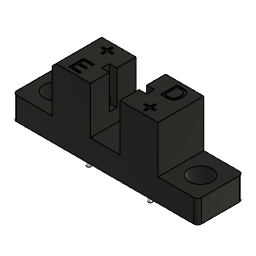
MOC7811 (Autodesk Fusion 360 design; units mm, degrees)
Autodesk Fusion 360 part; units mm, degrees
sketch "Sketch2" plane through (0, 0, 0) normal (0, 1, 0) x (1, 0, 0)
  line L0 (0, 0) -> (24.3, 0)
  line L1 (24.3, 0) -> (24.3, -3)
  line L2 (24.3, -3) -> (19.1, -3)
  line L3 (19.1, -3) -> (19.1, -9.2)
  line L4 (19.1, -9.2) -> (14.1, -9.2)
  line L5 (14.1, -9.2) -> (14.1, -3)
  line L6 (14.1, -3) -> (10.2, -3)
  line L7 (10.2, -3) -> (10.2, -9.2)
  line L8 (10.2, -9.2) -> (5.2, -9.2)
  line L9 (5.2, -9.2) -> (5.2, -3)
  line L10 (5.2, -3) -> (0, -3)
  line L11 (0, -3) -> (0, 0)
  dimension "d1" = 24.3
  dimension "d2" = 3
  dimension "d4" = 6.2
  dimension "d5" = 5
  dimension "d6" = 6.2
  dimension "d7" = 3.9
  dimension "d8" = 6.2
  dimension "d9" = 5
  dimension "d10" = 6.2
  constraint coincident L0.start L11.end
  constraint horizontal L0
  constraint perpendicular L0 L1
  constraint perpendicular L1 L2
  constraint perpendicular L2 L3
  constraint perpendicular L3 L4
  constraint perpendicular L4 L5
  constraint perpendicular L5 L6
  constraint perpendicular L6 L7
  constraint perpendicular L7 L8
  constraint perpendicular L8 L9
  constraint perpendicular L7 L10
  constraint perpendicular L0 L11
  constraint equal L2 L10
  measures "d1" distance of L0.start L0.end
  measures "d2" distance of L0.end L1.end
  measures "d4" distance of L2.end L3.end
  measures "d5" distance of L3.end L4.end
  measures "d6" distance of L4.end L5.end
  measures "d7" distance of L5.end L6.end
  measures "d8" distance of L6.end L7.end
  measures "d9" distance of L7.end L8.end
  measures "d10" distance of L8.end L9.end
extrude "Extrude1" add sketch "Sketch2" along normal blind 6
sketch "Sketch3" plane through (0, 0, 3) normal (0, 0, 1) x (-1, 0, 0)
  line L0 (0, 0) -> (-5.2, 0)
  line L1 (-5.2, 0) -> (-5.2, -6)
  line L2 (-5.2, -6) -> (0, -6)
  line L3 (0, -6) -> (0, 0)
  line L4 (-5.2, -6) -> (0, 0) construction
  line L5 (-5.2, 0) -> (0, -6) construction
  circle A0 centre (-2.6, -3) radius 1.5
  dimension "d13" = 3
  constraint coincident L1.end L2.start
  constraint coincident L0.start L3.end
  constraint coincident L0.end L1.start
  constraint coincident L2.end L3.start
  constraint midpoint L4 A0.centre
  measures "d13" diameter of A0
extrude "Extrude2" cut sketch "Sketch3" against normal blind 3 contours A0
sketch "Sketch4" plane through (0, 0, 3) normal (0, 0, 1) x (-1, 0, 0)
  line L0 (-19.1, 0) -> (-24.3, 0)
  line L1 (-24.3, 0) -> (-24.3, -6)
  line L2 (-24.3, -6) -> (-19.1, -6)
  line L3 (-19.1, -6) -> (-19.1, 0)
  line L4 (-19.1, -6) -> (-24.3, 0) construction
  line L5 (-24.3, -6) -> (-19.1, 0) construction
  circle A0 centre (-21.7, -3) radius 1.5
  dimension "d16" = 3
  constraint coincident L2.end L3.start
  constraint coincident L0.end L1.start
  constraint coincident L1.end L2.start
  constraint coincident L0.start L3.end
  constraint midpoint L4 A0.centre
  measures "d16" diameter of A0
extrude "Extrude3" cut sketch "Sketch4" against normal blind 3 contours A0
chamfer "Chamfer1" distance 0.5 angle 45 1 edges at (5.2, 3, 9.2)
sketch "Sketch5" plane through (10.2, 0, 0) normal (1, 0, 0) x (0, 1, 0)
  line L0 (0, 9.2) -> (0, 3)
  line L1 (0, 3) -> (6, 3)
  line L2 (6, 3) -> (6, 9.2)
  line L3 (6, 9.2) -> (0, 9.2)
fillet "Fillet1" radius 0.5 2 edges at (0, 6, 1.5) (0, 0, 1.5)
fillet "Fillet2" radius 0.5 2 edges at (24.3, 0, 1.5) (24.3, 6, 1.5)
sketch "Sketch7" plane through (0, 0, 9.2) normal (0, 0, 1) x (-1, 0, 0)
  line L0 (-5.7, -6) -> (-5.7, 0)
  line L1 (-5.7, 0) -> (-10.2, 0)
  line L2 (-10.2, 0) -> (-10.2, -6)
  line L3 (-10.2, -6) -> (-5.7, -6)
  line L4 (-11.2, -2.5) -> (-9.2, -2.5)
  line L5 (-9.2, -2.5) -> (-9.2, -3.5)
  line L6 (-9.2, -3.5) -> (-11.2, -3.5)
  line L7 (-11.2, -3.5) -> (-11.2, -2.5)
  line L8 (-11.2, -2.5) -> (-9.2, -3.5) construction
  line L9 (-9.2, -2.5) -> (-11.2, -3.5) construction
  point P0 (-10.2, -3)
  dimension "d22" = 2
  dimension "d23" = 1
  constraint horizontal L4
  constraint perpendicular L4 L5
  constraint parallel L4 L6
  constraint parallel L5 L7
  constraint coincident L8 P0
  constraint coincident L9 P0
  constraint midpoint L2 P0
  measures "d22" distance of L5.end L6.end
  measures "d23" distance of L4.end L5.end
extrude "Extrude4" cut sketch "Sketch7" against normal blind 4.5 contours L2 L4 L5 L6
ref_plane "WorkPlane1" through (12.15, 3, 5.85) normal (-1, 0, 0) x (0, 0, 1)
mirror "Mirror1" about plane through (12.15, 3, 5.85) normal (-1, 0, 0) of 4 faces at (9.5333, 3.5, 7.7) (9.2, 2.8333, 7.7) (9.8667, 2.5, 7.7) (9.5333, 3.1667, 4.7)
sketch "Sketch8" plane through (0, 0, 0) normal (0, 0, -1) x (1, 0, 0)
  arc A0 (23.8, -6) -> (24.3, -5.5) centre (23.8, -5.5) ccw
  line L0 (24.3, -5.5) -> (24.3, -0.5)
  arc A1 (24.3, -0.5) -> (23.8, 0) centre (23.8, -0.5) ccw
  line L1 (23.8, 0) -> (0.5, 0)
  arc A2 (0.5, 0) -> (0, -0.5) centre (0.5, -0.5) ccw
  line L2 (0, -0.5) -> (0, -5.5)
  arc A3 (0, -5.5) -> (0.5, -6) centre (0.5, -5.5) ccw
  line L3 (0.5, -6) -> (23.8, -6)
  circle A4 centre (21.7, -3) radius 1.5
  circle A5 centre (2.6, -3) radius 1.5
  line L4 (17.3061, -5.5) -> (7.3061, -5.5)
  line L5 (7.3061, -5.5) -> (7.3061, -0.5)
  line L6 (7.3061, -0.5) -> (17.3061, -0.5)
  line L7 (17.3061, -0.5) -> (17.3061, -5.5)
  line L8 (17.3061, -5.5) -> (7.3061, -0.5) construction
  line L9 (7.3061, -5.5) -> (17.3061, -0.5) construction
  point P0 (12.3061, -3)
  dimension "d27" = 10
  dimension "d28" = 5
  constraint horizontal L4
  constraint perpendicular L4 L5
  constraint parallel L4 L6
  constraint parallel L5 L7
  constraint coincident L8 P0
  constraint coincident L9 P0
  measures "d27" distance of L5.end L6.end
  measures "d28" distance of L4.end L5.end
extrude "Extrude5" cut sketch "Sketch8" against normal blind 2 contours L4 L5 L6 L7
sketch "Sketch9" plane through (0, 0, 2) normal (0, 0, -1) x (1, 0, 0)
  line L0 (17.3061, -0.5) -> (7.3061, -0.5)
  line L1 (7.3061, -0.5) -> (7.3061, -5.5)
  line L2 (7.3061, -5.5) -> (17.3061, -5.5)
  line L3 (17.3061, -5.5) -> (17.3061, -0.5)
  line L4 (7.3061, -0.5) -> (9.3061, -0.5)
  line L5 (9.3061, -0.5) -> (9.3061, -5.5)
  line L6 (9.3061, -5.5) -> (7.3061, -5.5)
  line L7 (7.3061, -5.5) -> (7.3061, -0.5)
  line L8 (17.3061, -0.5) -> (15.3061, -0.5)
  line L9 (15.3061, -0.5) -> (15.3061, -6)
  line L10 (15.3061, -6) -> (17.3061, -6)
  line L11 (17.3061, -6) -> (17.3061, -0.5)
  dimension "d31" = 2
  dimension "d32" = 2
  constraint horizontal L4
  constraint vertical L5
  constraint horizontal L6
  constraint vertical L7
  constraint coincident L0.end L1.start
  constraint horizontal L8
  constraint vertical L9
  constraint horizontal L10
  constraint vertical L11
  constraint coincident L0.start L3.end
  measures "d31" distance of L0.end L4.end
  measures "d32" distance of L0.start L8.end
extrude "Extrude6" cut sketch "Sketch9" against normal blind 3.5 contours L0 L2 L3 L8 L9 L11 | L0 L1 L2 L4 L5 L6 L7
sketch "Sketch10" plane through (0, 0, 5.5) normal (0, 0, -1) x (1, 0, 0)
  line L0 (9.3061, -3.5) -> (9.2, -3.5)
  line L1 (9.2, -3.5) -> (9.2, -2.5)
  line L2 (9.2, -2.5) -> (9.3061, -2.5)
  line L3 (9.3061, -2.5) -> (9.3061, -0.5)
  line L4 (9.3061, -0.5) -> (7.3061, -0.5)
  line L5 (7.3061, -0.5) -> (7.3061, -5.5)
  line L6 (7.3061, -5.5) -> (9.3061, -5.5)
  line L7 (9.3061, -5.5) -> (9.3061, -3.5)
  line L8 (9.2, -3) -> (7.3061, -3)
  line L9 (8.2531, -3) -> (8.2531, -1.73)
  circle A0 centre (8.2531, -1.73) radius 0.25
  circle A1 centre (8.2531, -4.27) radius 0.25
  line L10 (9.3061, -0.5) -> (9.3061, -5.5)
  line L11 (9.3061, -5.5) -> (15.3061, -5.5)
  line L12 (15.3061, -5.5) -> (15.3061, -0.5)
  line L13 (15.3061, -0.5) -> (9.3061, -0.5)
  line L14 (12.3061, -0.5) -> (12.3061, -2.7714)
  circle A2 centre (16.3592, -1.73) radius 0.25
  circle A3 centre (16.3592, -4.27) radius 0.25
  dimension "d35" = 1.27
  dimension "d37" = 0.5
  constraint midpoint L1 L8.start
  constraint midpoint L5 L8.end
  constraint midpoint L8 L9.start
  constraint perpendicular L8 L9
  constraint coincident L9.end A0.centre
  constraint symmetric L8 A0 A1
  constraint midpoint L13 L14.start
  constraint perpendicular L13 L14
  constraint symmetric A0 L14 A2
  constraint symmetric A1 L14 A3
  measures "d35" distance of L9.start L9.end
  measures "d37" diameter of A0
extrude "Extrude7" add sketch "Sketch10" along normal blind 7.5 contours A0 | A1 | A2 | A3
sketch "Sketch11" plane through (0, 0, 9.2) normal (0, 0, 1) x (-1, 0, 0)
  line L0 (-5.7, -6) -> (-5.7, 0)
  line L1 (-5.7, 0) -> (-10.2, 0)
  line L2 (-10.2, 0) -> (-10.2, -2.5)
  line L3 (-10.2, -2.5) -> (-9.2, -2.5)
  line L4 (-9.2, -2.5) -> (-9.2, -3.5)
  line L5 (-9.2, -3.5) -> (-10.2, -3.5)
  line L6 (-10.2, -3.5) -> (-10.2, -6)
  line L7 (-10.2, -6) -> (-5.7, -6)
  line L8 (-6.902, -0.4591) -> (-8.354, -0.4591) construction
  line L9 (-8.354, -0.4591) -> (-8.354, -3.1774) construction
  line L10 (-8.354, -3.1774) -> (-6.902, -3.1774) construction
  line L11 (-6.902, -3.1774) -> (-6.902, -0.4591) construction
  line L12 (-6.8464, -4.155) -> (-8.2644, -4.155) construction
  line L13 (-8.2644, -4.155) -> (-8.2644, -7.155) construction
  line L14 (-8.2644, -7.155) -> (-6.8464, -7.155) construction
  line L15 (-6.8464, -7.155) -> (-6.8464, -4.155) construction
  text T0 "E" font "Arial" height 2.7183 align ink ink in box 0 x 0 at (-6.902, -0.4591) x (-1, 0) y (0, -1) spacing 1 height is em
  text T1 "+" font "Arial" height 3 align ink ink in box 0 x 0 at (-6.8464, -4.155) x (-1, 0) y (0, -1) spacing 1 height is em
  constraint perpendicular L8 L9
  constraint parallel L8 L10
  constraint parallel L9 L11
  constraint perpendicular L12 L13
  constraint parallel L12 L14
  constraint parallel L13 L15
extrude "Extrude8" cut sketch "Sketch11" against normal blind 0.1 text T0 T1
sketch "Sketch12" plane through (0, 0, 9.2) normal (0, 0, 1) x (-1, 0, 0)
  line L0 (-15.1, -2.5) -> (-14.1, -2.5)
  line L1 (-14.1, -2.5) -> (-14.1, 0)
  line L2 (-14.1, 0) -> (-19.1, 0)
  line L3 (-19.1, 0) -> (-19.1, -6)
  line L4 (-19.1, -6) -> (-14.1, -6)
  line L5 (-14.1, -6) -> (-14.1, -3.5)
  line L6 (-14.1, -3.5) -> (-15.1, -3.5)
  line L7 (-15.1, -3.5) -> (-15.1, -2.5)
  line L8 (-16.0683, -3.3604) -> (-17.8437, -3.3604) construction
  line L9 (-17.8437, -3.3604) -> (-17.8437, -6.3604) construction
  line L10 (-17.8437, -6.3604) -> (-16.0683, -6.3604) construction
  line L11 (-16.0683, -6.3604) -> (-16.0683, -3.3604) construction
  line L12 (-16.1259, -1.9204) -> (-16.1259, -0.5025) construction
  line L13 (-16.1259, -0.5025) -> (-19.1259, -0.5025) construction
  line L14 (-19.1259, -0.5025) -> (-19.1259, -1.9204) construction
  line L15 (-19.1259, -1.9204) -> (-16.1259, -1.9204) construction
  text T0 "D" font "Arial" height 3 align ink ink in box 0 x 0 at (-16.0683, -3.3604) x (-1, 0) y (0, -1) spacing 1 height is em
  text T1 "+" font "Arial" height 3 align ink ink in box 0 x 0 at (-16.1259, -1.9204) x (0, 1) y (-1, 0) spacing 1 height is em
  constraint perpendicular L8 L9
  constraint parallel L8 L10
  constraint parallel L9 L11
  constraint perpendicular L12 L13
  constraint parallel L12 L14
  constraint parallel L13 L15
extrude "Extrude9" cut sketch "Sketch12" against normal blind 0.1 text T0 T1
sketch "Sketch13" plane through (0, 0, 0) normal (0, 0, -1) x (1, 0, 0)
  line L0 (7.3061, -5.5) -> (7.3061, -0.5)
  line L1 (7.3061, -0.5) -> (17.3061, -0.5)
  line L2 (17.3061, -0.5) -> (17.3061, -5.5)
  line L3 (17.3061, -5.5) -> (7.3061, -5.5)
  arc A0 (23.8, -6) -> (24.3, -5.5) centre (23.8, -5.5) ccw
  line L4 (24.3, -5.5) -> (24.3, -0.5)
  arc A1 (24.3, -0.5) -> (23.8, 0) centre (23.8, -0.5) ccw
  line L5 (23.8, 0) -> (0.5, 0)
  arc A2 (0.5, 0) -> (0, -0.5) centre (0.5, -0.5) ccw
  line L6 (0, -0.5) -> (0, -5.5)
  arc A3 (0, -5.5) -> (0.5, -6) centre (0.5, -5.5) ccw
  line L7 (0.5, -6) -> (23.8, -6)
  circle A4 centre (21.7, -3) radius 1.5
  circle A5 centre (2.6, -3) radius 1.5
  line L8 (8.3061, -4) -> (6.3061, -4)
  line L9 (6.3061, -4) -> (6.3061, -2)
  line L10 (6.3061, -2) -> (8.3061, -2)
  line L11 (8.3061, -2) -> (8.3061, -4)
  line L12 (8.3061, -4) -> (6.3061, -2) construction
  line L13 (6.3061, -4) -> (8.3061, -2) construction
  line L14 (18.3061, -4) -> (18.3061, -2)
  line L15 (18.3061, -2) -> (16.3061, -2)
  line L16 (16.3061, -4) -> (18.3061, -4)
  line L17 (16.3061, -2) -> (16.3061, -4)
  point P0 (7.3061, -3)
  dimension "d44" = 2
  dimension "d45" = 2
  constraint horizontal L8
  constraint perpendicular L8 L9
  constraint parallel L8 L10
  constraint parallel L9 L11
  constraint coincident L12 P0
  constraint coincident L13 P0
  constraint midpoint L0 P0
  measures "d44" distance of L9.end L10.end
  measures "d45" distance of L8.end L9.end
extrude "Extrude10" cut sketch "Sketch13" against normal blind 0.1 contours L0 L8 L9 L10 | L2 L14 L15 L16
equation "d35 = ( 2.54 / 2 ) * 1 mm"
equation "d38 = 5.50 mm + 2 mm"
